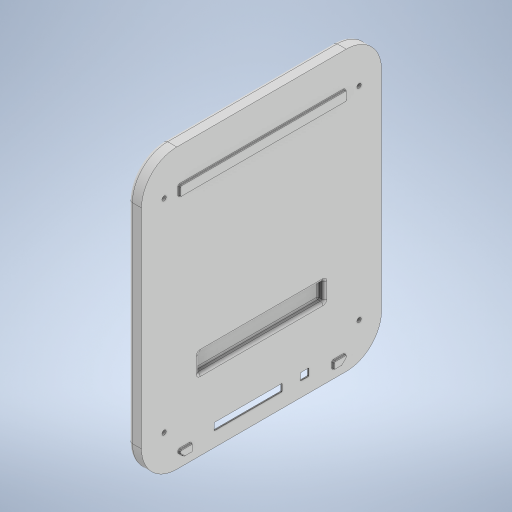
# Autodesk Inventor part: BacklightCaseBack
Saved by Autodesk Inventor 2023 (Build 270158000, 158)
## iProperties
Created: 2026-01-31
Part Number: BacklightCaseBack
Material: Generic
Document SubType Name: Modeling
Designer: DanAr
Density: 1 g/cm^3
Appearance: Default
Author: DanAr
Autodesk Inventor part; units mm, degrees
ref_plane "YZ Plane" through (0, 0, 0) normal (1, 0, 0) x (0, 1, 0)
ref_plane "XZ Plane" through (0, 0, 0) normal (0, 1, 0) x (-1, 0, 0)
ref_plane "XY Plane" through (0, 0, 0) normal (0, 0, 1) x (1, 0, 0)
sketch "Sketch1" plane through (0, 0, 0) normal (1, 0, 0) x (0, 1, 0)
  line L0 (0, 0) -> (214, 0)
  line L1 (214, 0) -> (214, -184)
  line L2 (214, -184) -> (0, -184)
  line L3 (0, -184) -> (0, 0)
  line L4 (214, -92) -> (0, -92)
  line L5 (29.25, -166.75) -> (184.75, -166.75)
  line L6 (184.75, -166.75) -> (184.75, -17.25)
  line L7 (184.75, -17.25) -> (29.25, -17.25)
  line L8 (29.25, -17.25) -> (29.25, -166.75)
  line L9 (29.25, -166.75) -> (184.75, -17.25) construction
  line L10 (184.75, -166.75) -> (29.25, -17.25) construction
  circle A0 centre (184.75, -17.25) radius 1.6
  circle A1 centre (184.75, -166.75) radius 1.6
  circle A2 centre (29.25, -17.25) radius 1.6
  circle A3 centre (29.25, -166.75) radius 1.6
  point P0 (107, -92)
  dimension "d0" = 184
  dimension "d1" = 214
  dimension "d2" = 17.25
  dimension "d3" = 29.25
  dimension "d4" = 3.2
  constraints: 22 end point, 5 midpoint, 4 centre point, 4 coincident, 4 parallel, 2 horizontal, 2 perpendicular
  measures "d0" distance of L0.end L1.end
  measures "d1" distance of L1.end L2.end
  measures "d2" distance between parallel lines of L0 L7
  measures "d3" distance between parallel lines of L1 L6
  measures "d4" diameter of A0
extrude "Extrusion1" add sketch "Sketch1" along normal blind 10 contours L0 L1 L4 L6 A0 L7 A2 L8 L3 | L4 L8 A3 L5 A1 L6 L1 L2 L3 | L8 A2 L7 A0 L6 L4 | L4 L6 A1 L5 A3 L8
fillet "Fillet1" radius 27 4 edges at (5, 214, 0) (5, 214, -184) (5, 0, 0) (5, 0, -184)
sketch "Sketch2" plane through (10, 0, 0) normal (1, 0, 0) x (0, 0, -1)
  line L0 (27, 0) -> (157, 0) projected
  line L1 (92, 0) -> (92, 97.6)
  line L2 (27.9, 188.6) -> (156.1, 188.6)
  line L3 (156.1, 188.6) -> (156.1, 6.6)
  line L4 (156.1, 6.6) -> (27.9, 6.6)
  line L5 (27.9, 6.6) -> (27.9, 188.6)
  line L6 (27.9, 188.6) -> (156.1, 6.6) construction
  line L7 (156.1, 188.6) -> (27.9, 6.6) construction
  point P0 (0, 0)
  dimension "d8" = 97.6
  dimension "d9" = 182
  dimension "d10" = 128.2
  constraints: 14 end point, 3 midpoint, 2 parallel, 1 horizontal, 1 perpendicular, 1 vertical
  measures "d8" distance of L1.start L1.end
  measures "d9" distance of L2.end L3.end
  measures "d10" distance of L2.start L2.end
extrude "Extrusion2" cut sketch "Sketch2" against normal blind 5
chamfer "Chamfer1" distance 4 angle 45 2 edges at (7.5, 6.6, -156.1) (7.5, 6.6, -27.9)
sketch "Sketch3" plane through (5, 0, 0) normal (1, 0, 0) x (0, 0, -1)
  line L0 (152.1, 6.6) -> (31.9, 6.6) projected
  line L1 (156.1, 188.6) -> (156.1, 10.6) projected
  line L2 (152.1, 6.6) -> (156.1, 6.6)
  line L3 (156.1, 6.6) -> (156.1, 10.6)
  line L4 (156.1, 10.6) -> (152.1, 10.6)
  line L5 (152.1, 10.6) -> (152.1, 6.6)
  line L6 (156.1, 6.6) -> (96.1, 6.6)
  line L7 (96.1, 6.6) -> (96.1, 68.6)
  line L8 (96.1, 68.6) -> (156.1, 68.6)
  line L9 (156.1, 68.6) -> (156.1, 6.6)
  line L10 (96.1, 68.6) -> (140.1, 68.6)
  line L11 (140.1, 68.6) -> (140.1, 54.6)
  line L12 (140.1, 54.6) -> (96.1, 54.6)
  line L13 (96.1, 54.6) -> (96.1, 68.6)
  line L14 (27.9, 188.6) -> (156.1, 188.6) projected
  line L15 (27.9, 188.6) -> (156.1, 188.6)
  line L16 (156.1, 188.6) -> (156.1, 6.6)
  line L17 (156.1, 6.6) -> (27.9, 6.6)
  line L18 (27.9, 6.6) -> (27.9, 188.6)
  line L19 (96.1, 54.6) -> (43.9, 54.6)
  line L20 (43.9, 54.6) -> (43.9, 68.6)
  line L21 (43.9, 68.6) -> (96.1, 68.6)
  line L22 (96.1, 68.6) -> (96.1, 54.6)
  point P0 (0, 0)
  point P1 (31.9, 6.6)
  dimension "d16" = 60
  dimension "d17" = 62
  dimension "d18" = 14
  dimension "d19" = 44
  dimension "d40" = 52.2
  constraints: 40 end point, 10 parallel, 5 horizontal, 5 perpendicular
  measures "d16" distance of L7.end L8.end
  measures "d17" distance of L6.end L7.end
  measures "d18" distance of L10.end L11.end
  measures "d19" distance of L11.end L12.end
  measures "d40" distance of L12.end L19.end
extrude "Extrusion3" add sketch "Sketch3" along normal blind 4 contours L5 L4 L3 L2 | L0 L7 L12 L11 L8 L1 L4 L5 | L0 L17 L18 L14 L1 L8 L21 L20 L19 L7
sketch "Sketch4" plane through (9, 0, 0) normal (1, 0, 0) x (0, 0, -1)
  line L0 (27.9, 10.6) -> (31.9, 6.6) projected
  line L1 (37.9, -3.4) -> (37.9, 12.6)
  line L2 (37.9, 12.6) -> (27.9, 12.6)
  line L3 (27.9, 12.6) -> (27.9, 10.6)
  line L4 (27.9, -3.4) -> (27.9, -7.4)
  line L5 (37.9, -7.4) -> (37.9, -3.4)
  line L6 (152.1, 6.6) -> (31.9, 6.6) projected
  line L7 (37.9, 12.6) -> (146.1, 12.6)
  line L8 (146.1, 12.6) -> (146.1, 6.6)
  line L9 (146.1, 6.6) -> (37.9, 6.6)
  line L10 (37.9, 6.6) -> (37.9, 12.6)
  line L11 (146.1, 12.6) -> (156.1, 12.6)
  line L12 (156.1, 12.6) -> (156.1, 6.6)
  line L13 (156.1, 6.6) -> (146.1, 6.6)
  line L14 (146.1, 6.6) -> (146.1, 12.6)
  line L15 (152.1, 6.6) -> (156.1, 10.6) projected
  line L16 (156.1, 10.6) -> (152.1, 6.6)
  point P0 (0, 0)
  point P1 (37.9, 6.6)
  dimension "d22" = 10
  dimension "d23" = 2
  dimension "d24" = 10
  dimension "d25" = 108.2
  constraints: 28 end point, 6 parallel, 2 horizontal, 2 perpendicular, 2 point on line, 1 collinear, 2 other
  measures "d22" distance of L1.end L2.end
  measures "d23" distance of L2.end L0.start
  measures "d24" distance of L7.end L11.end
  measures "d25" distance of L1.end L7.end
extrude "Extrusion4" add sketch "Sketch4" along normal blind 2.5 contours L3 L2 L1 L6 L0 | L8 L11 L12 L15 L6 | L15 L12 L13
sketch "Sketch5" plane through (9, 0, 0) normal (1, 0, 0) x (0, 0, -1)
  line L0 (27.9, 188.6) -> (156.1, 188.6) projected
  line L1 (156.1, 188.6) -> (156.1, 12.6) projected
  line L2 (27.9, 188.6) -> (156.1, 188.6)
  line L3 (156.1, 188.6) -> (156.1, 180.6)
  line L4 (156.1, 180.6) -> (27.9, 180.6)
  line L5 (27.9, 180.6) -> (27.9, 188.6)
  point P0 (0, 0)
  dimension "d28" = 8
  constraints: 8 end point, 2 parallel, 1 horizontal, 1 perpendicular, 1 point on line
  measures "d28" distance between parallel lines of L0 L4
extrude "Extrusion5" add sketch "Sketch5" along normal blind 2.5
chamfer "Chamfer3" distance 4.3 angle 45 1 edges at (10.75, 6.6, -156.1)
sketch "Sketch7" plane through (11.5, 0, 0) normal (1, 0, 0) x (0, 0, -1)
  line L0 (156.1, 188.6) -> (27.9, 188.6) projected
  line L1 (27.9, 172.6) -> (156.1, 172.6)
  line L2 (156.1, 172.6) -> (156.1, 188.6)
  line L3 (156.1, 188.6) -> (27.9, 188.6)
  line L4 (27.9, 188.6) -> (27.9, 172.6)
  line L5 (27.9, 180.6) -> (156.1, 180.6) projected
  line L6 (27.9, 172.6) -> (156.1, 188.6) construction
  line L7 (156.1, 172.6) -> (27.9, 188.6) construction
  line L8 (28.2, 172.9) -> (155.8, 172.9)
  line L9 (155.8, 172.9) -> (155.8, 188.3)
  line L10 (155.8, 188.3) -> (28.2, 188.3)
  line L11 (28.2, 188.3) -> (28.2, 172.9)
  line L12 (28.2, 172.9) -> (155.8, 188.3) construction
  line L13 (155.8, 172.9) -> (28.2, 188.3) construction
  line L14 (27.9, 12.6) -> (37.9, 12.6) projected
  line L15 (27.9, 12.6) -> (156.1, 12.6)
  line L16 (28.2, 18.3) -> (155.8, 18.3)
  line L17 (155.8, 18.3) -> (155.8, 6.9)
  line L18 (155.8, 6.9) -> (28.2, 6.9)
  line L19 (28.2, 6.9) -> (28.2, 18.3)
  line L20 (28.2, 18.3) -> (155.8, 6.9) construction
  line L21 (155.8, 18.3) -> (28.2, 6.9) construction
  line L22 (156.8837, 19.0304) -> (27.1163, 19.0304)
  line L23 (27.1163, 19.0304) -> (27.1163, 6.1696)
  line L24 (27.1163, 6.1696) -> (156.8837, 6.1696)
  line L25 (156.8837, 6.1696) -> (156.8837, 19.0304)
  line L26 (156.8837, 19.0304) -> (27.1163, 6.1696) construction
  line L27 (27.1163, 19.0304) -> (156.8837, 6.1696) construction
  point P0 (0, 0)
  point P1 (92, 180.6)
  point P2 (92, 180.6)
  point P3 (92, 12.6)
  point P4 (155.8, 180.6)
  point P5 (28.2, 180.6)
  dimension "d41" = 127.6
  dimension "d42" = 15.4
  dimension "d43" = 11.4
  dimension "d44" = 127.6
  constraints: 50 end point, 11 midpoint, 8 parallel, 5 horizontal, 4 perpendicular
  measures "d41" distance of L9.end L10.end
  measures "d42" distance of L8.end L9.end
  measures "d43" distance of L16.end L17.end
  measures "d44" distance of L17.end L18.end
extrude "Extrusion7" cut sketch "Sketch7" against normal up to surface (1.5 mm away) contours L2 L5 L9 L10 L11 L4 L0 | L25 L24 L23 L22
fillet "Fillet2" radius 1 6 edges at (10.75, 188.3, -155.8) (10.75, 188.3, -28.2) (10.75, 10.3, -28.2) (10.75, 6.9, -31.6) (10.75, 10.6, -155.8) (10.75, 6.9, -152.1)
sketch "Sketch8" plane through (9, 0, 0) normal (1, 0, 0) x (0, 0, -1)
  line L0 (146.1, 6.6) -> (37.9, 6.6) projected
  line L1 (154.8, 188.3) -> (29.2, 188.3) projected
  line L2 (146.1, 6.6) -> (37.9, 6.6) projected
  line L3 (37.9, 6.6) -> (146.1, 6.6)
  line L4 (146.1, 6.6) -> (146.1, 92.3)
  line L5 (146.1, 92.3) -> (37.9, 92.3)
  line L6 (37.9, 92.3) -> (37.9, 6.6)
  line L7 (56, 173.3) -> (128, 173.3)
  line L8 (128, 173.3) -> (128, 11.3)
  line L9 (128, 11.3) -> (56, 11.3)
  line L10 (56, 11.3) -> (56, 173.3)
  line L11 (56, 173.3) -> (128, 11.3) construction
  line L12 (128, 173.3) -> (56, 11.3) construction
  line L13 (56, 11.3) -> (107.5, 11.3)
  line L14 (107.5, 11.3) -> (107.5, 16.5)
  line L15 (107.5, 16.5) -> (56, 16.5)
  line L16 (56, 16.5) -> (56, 11.3)
  line L17 (128, 11.3) -> (122.2, 11.3)
  line L18 (122.2, 11.3) -> (122.2, 16.5)
  line L19 (122.2, 16.5) -> (128, 16.5)
  line L20 (128, 16.5) -> (128, 11.3)
  point P0 (0, 0)
  point P1 (92, 92.3)
  dimension "d48" = 181.7
  dimension "d49" = 85.7
  dimension "d50" = 162
  dimension "d51" = 72
  dimension "d52" = 51.5
  dimension "d53" = 5.2
  dimension "d54" = 5.8
  constraints: 36 end point, 8 parallel, 4 horizontal, 4 perpendicular, 3 midpoint
  measures "d48" distance between parallel lines of L0 L1
  measures "d49" distance of L5.end L0.end
  measures "d50" distance of L7.end L8.end
  measures "d51" distance of L8.end L9.end
  measures "d52" distance of L14.end L15.end
  measures "d53" distance of L13.end L14.end
  measures "d54" distance of L18.end L19.end
extrude "Extrusion8" cut sketch "Sketch8" against normal blind 10 contours L8 L9 L18 L19 | L15 L14 L9 L10
sketch "Sketch9" plane through (9, 0, 0) normal (1, 0, 0) x (0, 0, -1)
  line L0 (56, 16.5) -> (107.5, 16.5) projected
  line L1 (56, 11.3) -> (107.5, 11.3) projected
  line L2 (56, 16.5) -> (107.5, 16.5)
  line L3 (107.5, 16.5) -> (107.5, 11.3)
  line L4 (107.5, 11.3) -> (56, 11.3)
  line L5 (56, 11.3) -> (56, 16.5)
  line L6 (122.2, 11.3) -> (122.2, 16.5) projected
  line L7 (128, 11.3) -> (128, 16.5) projected
  line L8 (122.2, 11.3) -> (128, 11.3)
  line L9 (128, 11.3) -> (128, 16.5)
  line L10 (128, 16.5) -> (122.2, 16.5)
  line L11 (122.2, 16.5) -> (122.2, 11.3)
  line L12 (43.9, 54.6) -> (140.1, 54.6) projected
  line L13 (43.9, 68.6) -> (140.1, 68.6) projected
  line L14 (43.9, 54.6) -> (140.1, 54.6)
  line L15 (140.1, 54.6) -> (140.1, 68.6)
  line L16 (140.1, 68.6) -> (43.9, 68.6)
  line L17 (43.9, 68.6) -> (43.9, 54.6)
  line L18 (27.9, 12.6) -> (27.9, 180.6) projected
  line L19 (27.9, 180.6) -> (156.1, 180.6)
  line L20 (156.1, 180.6) -> (156.1, 6.5301)
  line L21 (156.1, 6.5301) -> (27.9, 6.5301)
  line L22 (27.9, 6.5301) -> (27.9, 180.6)
  point P0 (0, 0)
  constraints: 32 end point, 8 parallel, 4 horizontal, 4 perpendicular
extrude "Extrusion9" add sketch "Sketch9" along normal up to surface (1 mm away)
sketch "Sketch11" plane through (0, 0, 0) normal (-1, 0, 0) x (0, 0, 1)
  line L0 (-147.8827, -27.8) -> (-36.1173, -27.8)
  line L1 (-36.1173, -27.8) -> (-36.1173, 27.8)
  line L2 (-36.1173, 27.8) -> (-147.8827, 27.8)
  line L3 (-147.8827, 27.8) -> (-147.8827, -27.8)
  line L4 (-27, 0) -> (-157, 0) projected
  line L5 (-147.8827, -27.8) -> (-36.1173, 27.8) construction
  line L6 (-36.1173, -27.8) -> (-147.8827, 27.8) construction
  point P0 (0, 0)
  point P1 (-92, 0)
  point P2 (-147.8827, 0)
  point P3 (-36.1173, 0)
  dimension "d59" = 55.6
  constraints: 12 end point, 3 midpoint, 2 parallel, 1 horizontal, 1 perpendicular
  measures "d59" distance of L0.end L1.end
extrude "Extrusion10" cut sketch "Sketch11" against normal blind 9 contours L3 L2 L1 L4
fillet "Fillet3" radius 13.5 2 edges at (4.5, 27.8, -147.8827) (4.5, 27.8, -36.1173)
fillet "Fillet4" radius 4 2 edges at (4.5, 0, -147.8827) (4.5, 0, -36.1173)
fillet "Fillet5" radius 4 7 edges at (9, 23.8459, -143.9286) (9, 9.15, -147.8827) (9, 1.1716, -149.0543) (9, 27.8, -92) (9, 23.8459, -40.0714) (9, 9.15, -36.1173) (9, 1.1716, -34.9457)
fillet "Fillet6" radius 0.8 5 edges at (9, 0, -92) (6.7765, 0, -150.0112) (8.7951, 0, -146.4628) (8.7951, 0, -37.5372) (6.7765, 0, -33.9888)
fillet "Fillet7" radius 3 16 edges at (0, 27.8, -92) (0, 23.8459, -40.0714) (0, 9.15, -36.1173) (0, 1.1716, -34.9457) (0, 0, -29.5586) (0, 7.9081, -7.9081) (0, 107, 0) (0, 206.0919, -7.9081) (0, 214, -92) (0, 206.0919, -176.0919) (0, 107, -184) (0, 7.9081, -176.0919) (0, 0, -154.4414) (0, 1.1716, -149.0543) (0, 9.15, -147.8827) (0, 23.8459, -143.9286)
sketch "Sketch12" plane through (0, 0, 0) normal (-1, 0, 0) x (0, 0, 1)
  circle A0 centre (-166.75, 184.75) radius 1.6 projected
  circle A1 centre (-166.75, 184.75) radius 2.6
  circle A2 centre (-17.25, 184.75) radius 1.6 projected
  circle A3 centre (-17.25, 184.75) radius 2.6
  circle A4 centre (-166.75, 29.25) radius 1.6 projected
  circle A5 centre (-166.75, 29.25) radius 2.6
  circle A6 centre (-17.25, 29.25) radius 1.6 projected
  circle A7 centre (-17.25, 29.25) radius 2.6
  point P0 (0, 0)
  dimension "d67" = 5.2
  constraints: 4 centre point, 4 coincident
  measures "d67" diameter of A1
extrude "Extrusion11" cut sketch "Sketch12" against normal blind 6 contours A0 | A1 | A2 | A3 | A4 | A5 | A6 | A7
chamfer "Chamfer4" distance 0.3 angle 45 4 edges at (6, 183.15, -166.75) (6, 183.15, -17.25) (6, 27.65, -166.75) (6, 27.65, -17.25)
fillet "Fillet8" radius 1 4 edges at (0, 184.75, -169.35) (0, 29.25, -169.35) (0, 29.25, -19.85) (0, 184.75, -19.85)
fillet "Fillet9" radius 0.1 8 edges at (9.5, 11.3, -128) (9.5, 11.3, -122.2) (9.5, 16.5, -122.2) (9.5, 16.5, -128) (9.5, 11.3, -107.5) (9.5, 16.5, -107.5) (9.5, 11.3, -56) (9.5, 16.5, -56)
fillet "Fillet10" radius 0.2 32 edges at (9, 11.3, -125.1) (9, 11.3293, -122.2293) (9, 13.9, -122.2) (9, 16.4707, -122.2293) (9, 16.5, -125.1) (9, 16.4707, -127.9707) (9, 13.9, -128) (9, 11.3293, -127.9707) (9, 11.3293, -56.0293) (9, 13.9, -56) (9, 16.4707, -56.0293) (9, 16.5, -81.75) (9, 16.4707, -107.4707) (9, 13.9, -107.5) (9, 11.3293, -107.4707) (9, 11.3, -81.75) (10, 11.3293, -127.9707) (10, 13.9, -128) (10, 16.4707, -127.9707) (10, 16.5, -125.1) (10, 16.4707, -122.2293) (10, 13.9, -122.2) (10, 11.3293, -122.2293) (10, 11.3, -125.1) (10, 11.3293, -107.4707) (10, 13.9, -107.5) (10, 16.4707, -107.4707) (10, 16.5, -81.75) (10, 16.4707, -56.0293) (10, 13.9, -56) (10, 11.3293, -56.0293) (10, 11.3, -81.75)
fillet "Fillet11" radius 1 4 edges at (7.5, 54.6, -140.1) (7.5, 68.6, -140.1) (7.5, 68.6, -43.9) (7.5, 54.6, -43.9)
fillet "Fillet12" radius 1 8 edges at (5, 54.6, -92) (5, 54.8929, -139.8071) (5, 61.6, -140.1) (5, 68.3071, -139.8071) (5, 68.6, -92) (5, 68.3071, -44.1929) (5, 61.6, -43.9) (5, 54.8929, -44.1929)
fillet "Fillet13" radius 2 8 edges at (10, 54.6, -92) (10, 54.8929, -139.8071) (10, 61.6, -140.1) (10, 68.3071, -139.8071) (10, 68.6, -92) (10, 68.3071, -44.1929) (10, 61.6, -43.9) (10, 54.8929, -44.1929)
fillet "Fillet14" radius 1 8 edges at (10.75, 12.6, -146.1) (10.75, 12.6, -155.8) (10.75, 6.9, -146.1) (10.75, 12.6, -28.2) (10.75, 6.9, -37.9) (10.75, 12.6, -37.9) (10.75, 180.6, -28.2) (10.75, 180.6, -155.8)
fillet "Fillet15" radius 0.4 56 edges at (10, 188.3, -92) (10, 188.0071, -28.4929) (10, 184.45, -28.2) (10, 180.8929, -28.4929) (10, 180.6, -92) (10, 180.8929, -155.5071) (10, 184.45, -155.8) (10, 188.0071, -155.5071) (10, 12.3071, -28.4929) (10, 11.1571, -28.2) (10, 10.3315, -28.2761) (10, 8.6, -29.9) (10, 6.9761, -31.6315) (10, 6.9, -34.4571) (10, 7.1929, -37.6071) (10, 9.75, -37.9) (10, 12.3071, -37.6071) (10, 12.6, -33.05) (10, 12.3071, -146.3929) (10, 9.75, -146.1) (10, 7.1929, -146.3929) (10, 6.9, -149.3929) (10, 6.9761, -152.0685) (10, 8.75, -153.95) (10, 10.6315, -155.7239) (10, 11.3071, -155.8) (10, 12.3071, -155.5071) (10, 12.6, -150.95) (11.5, 12.3071, -146.3929) (11.5, 9.75, -146.1) (11.5, 7.1929, -146.3929) (11.5, 6.9, -149.3929) (11.5, 6.9761, -152.0685) (11.5, 8.75, -153.95) (11.5, 10.6315, -155.7239) (11.5, 11.3071, -155.8) (11.5, 12.3071, -155.5071) (11.5, 12.6, -150.95) (11.5, 12.3071, -28.4929) (11.5, 11.1571, -28.2) (11.5, 10.3315, -28.2761) (11.5, 8.6, -29.9) (11.5, 6.9761, -31.6315) (11.5, 6.9, -34.4571) (11.5, 7.1929, -37.6071) (11.5, 9.75, -37.9) (11.5, 12.3071, -37.6071) (11.5, 12.6, -33.05) (11.5, 180.8929, -155.5071) (11.5, 184.45, -155.8) (11.5, 188.0071, -155.5071) (11.5, 188.3, -92) (11.5, 188.0071, -28.4929) (11.5, 184.45, -28.2) (11.5, 180.8929, -28.4929) (11.5, 180.6, -92)
sketch "Sketch13" plane through (0, 0, 0) normal (-1, 0, 0) x (0, 0, 1)
  line L0 (-144.5506, 0) -> (-39.4494, 0) projected
  line L1 (-134.3827, 27.8) -> (-49.6173, 27.8) projected
  line L2 (-36.1173, 14.3) -> (-36.1173, 4) projected
  line L3 (-147.8827, 4) -> (-147.8827, 14.3) projected
  line L4 (-184, 187) -> (-184, 27) projected
  line L5 (0, 27) -> (0, 187) projected
  line L6 (-122.3, 11.3) -> (-127.9, 11.3) projected
  line L7 (-128, 11.4) -> (-128, 16.4) projected
  line L8 (-56, 16.4) -> (-56, 11.4) projected
  line L9 (-56.1, 11.3) -> (-107.4, 11.3) projected
  line L10 (-107.4, 16.5) -> (-56.1, 16.5) projected
  line L11 (-122.2, 16.4) -> (-122.2, 11.4) projected
  line L12 (-107.5, 11.4) -> (-107.5, 16.4) projected
  point P0 (0, 0)
  point P1 (-92, 0)
  point P2 (-128, 13.9)
  point P3 (-107.5, 13.9)
  dimension "d81" = 27.8
  dimension "d82" = 111.7654
  dimension "d83" = 36.1173
  dimension "d84" = 36.1173
  dimension "d85" = 184
  dimension "d87" = 84.7654
  dimension "d88" = 11.3
  dimension "d89" = 19.8827
  dimension "d90" = 19.8827
  dimension "d91" = 72
  dimension "d92" = 5.2
  dimension "d93" = 14.7
  dimension "d94" = 13.9
  dimension "d95" = 5.8
  dimension "d96" = 51.5
  constraints: 3 midpoint
  measures "d81" distance from line of point (-92, 0) L1
  measures "d82" distance between parallel lines of L2 L3
  measures "d83" distance between parallel lines of L4 L3
  measures "d84" distance between parallel lines of L5 L2
  measures "d85" distance between parallel lines of L5 L4
  measures "d87" distance of L1.start L1.end
  measures "d88" distance between parallel lines of L0 L6
  measures "d89" distance from line of L3 point (-128, 13.9)
  measures "d90" distance between parallel lines of L2 L8
  measures "d91" distance between parallel lines of L8 L7
  measures "d92" distance between parallel lines of L9 L10
  measures "d93" distance between parallel lines of L11 L12
  measures "d94" distance from line of L0 point (-107.5, 13.9)
  measures "d95" distance between parallel lines of L7 L11
  measures "d96" distance between parallel lines of L8 L12
sketch "Sketch14" plane through (10, 27, 0) normal (0, 0, 1) x (1, 0, 0)
  line L0 (-10, 160) -> (-10, 0) projected
  line L1 (0, 160) -> (0, 0) projected
  point P0 (-10, -27)
  dimension "d86" = 10
  measures "d86" distance between parallel lines of L0 L1
body "Solid1"
